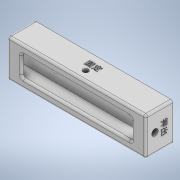
# Autodesk Inventor part: Part1
Saved by Autodesk Inventor 2021.4 (Build 254397000, 397)
## iProperties
Created: 2023-11-13
Part Number: Part1
Material: 一般
Document SubType Name: Modeling
Designer: ryusei
Density: 1 g/cm^3
Appearance: 既定
Author: ryusei
Autodesk Inventor part; units mm, degrees
ref_plane "YZ Plane" through (0, 0, 0) normal (1, 0, 0) x (0, 1, 0)
ref_plane "XZ Plane" through (0, 0, 0) normal (0, 1, 0) x (-1, 0, 0)
ref_plane "XY Plane" through (0, 0, 0) normal (0, 0, 1) x (1, 0, 0)
sketch "スケッチ1" plane through (0, 0, 0) normal (0, 0, 1) x (1, 0, 0)
  line L0 (-64, 17.5) -> (64, 17.5)
  line L1 (64, 17.5) -> (64, -17.5)
  line L2 (64, -17.5) -> (-64, -17.5)
  line L3 (-64, -17.5) -> (-64, 17.5)
  line L4 (-64, 17.5) -> (64, -17.5) construction
  line L5 (64, 17.5) -> (-64, -17.5) construction
  point P0 (0, 0)
  dimension "d0" = 128
  dimension "d1" = 35
  constraints: 12 end point, 2 midpoint, 2 parallel, 1 horizontal, 1 perpendicular
  measures "d0" distance of L1.end L2.end
  measures "d1" distance of L0.end L1.end
extrude "押し出し1" add sketch "スケッチ1" along normal blind 25
sketch "スケッチ3" plane through (-64, -17.5, 0) normal (-1, 0, 0) x (0, 0, 1)
  line L0 (10, 30) -> (23, 30)
  line L1 (23, 30) -> (23, 5)
  line L2 (23, 5) -> (10, 5)
  line L3 (10, 5) -> (10, 30)
  line L4 (0, 0) -> (25, 0) projected
  line L5 (25, 35) -> (25, 0) projected
  point P0 (0, 17.5)
  dimension "d8" = 13
  dimension "d9" = 25
  dimension "d10" = 5
  dimension "d11" = 2
  constraints: 8 end point, 2 parallel, 1 horizontal, 1 perpendicular
  measures "d8" distance of L1.end L2.end
  measures "d9" distance of L0.end L1.end
  measures "d10" distance between parallel lines of L4 L2
  measures "d11" distance between parallel lines of L5 L1
extrude "押し出し2" cut sketch "スケッチ3" against normal blind 118
sketch "スケッチ4" plane through (0, 0, 25) normal (0, 0, 1) x (1, 0, 0)
  line L0 (-51, 9.5) -> (51, 9.5)
  line L1 (51, 9.5) -> (51, -9.5)
  line L2 (51, -9.5) -> (-51, -9.5)
  line L3 (-51, -9.5) -> (-51, 9.5)
  line L4 (-51, 9.5) -> (51, -9.5) construction
  line L5 (51, 9.5) -> (-51, -9.5) construction
  point P0 (0, 0)
  dimension "d14" = 102
  dimension "d15" = 19
  constraints: 12 end point, 2 midpoint, 2 parallel, 1 horizontal, 1 perpendicular
  measures "d14" distance of L0.start L0.end
  measures "d15" distance of L0.end L1.end
extrude "押し出し3" cut sketch "スケッチ4" against normal blind 2
sketch "スケッチ6" plane through (64, -17.5, 0) normal (1, 0, 0) x (0, 0, -1)
  line L0 (0, 0) -> (-25, 0) projected
  line L1 (0, 0) -> (0, 35) projected
  line L2 (-25, 0) -> (-25, 35) projected
  point P0 (0, 17.5)
  point P1 (-16.5, 17.5)
  dimension "d27" = 17.5
  dimension "d46" = 8.5
  measures "d27" distance from line of L0 point (-16.5, 17.5)
  measures "d46" distance from line of L2 point (-16.5, 17.5)
hole "穴2" at (64, 0, 16.5) direction (-1, 0, 0) diameter 6 end through all
sketch "スケッチ7" plane through (-64, 17.5, 0) normal (0, 1, 0) x (1, 0, 0)
  line L0 (128, 0) -> (0, 0) projected
  line L1 (128, 0) -> (128, -25) projected
  line L2 (128, -25) -> (0, -25) projected
  point P0 (64, 0)
  point P1 (64, -16.5)
  dimension "d37" = 64
  dimension "d45" = 8.5
  measures "d37" distance from line of L1 point (64, -16.5)
  measures "d45" distance from line of L2 point (64, -16.5)
hole "穴3" at (0, 17.5, 16.5) direction (0, -1, 0) diameter 4.9 depth 8
sketch "スケッチ8" plane through (-64, -12.5, 10) normal (0, 0, 1) x (1, 0, 0)
  point P0 (64, 12.5)
  point P1 (29, 12.5)
  point P2 (99, 12.5)
  dimension "d47" = 35
  dimension "d48" = 35
  measures "d47" distance of point (29, 12.5) point (64, 12.5)
  measures "d48" distance of point (99, 12.5) point (64, 12.5)
hole "穴4" at (-35, 0, 10) at (35, 0, 10) direction (0, 0, -1) diameter 6 depth 15 counterbore diameter 10 counterbore depth 6
fillet "フィレット1" radius 2 12 edges at (-64, 17.5, 12.5) (0, 17.5, 25) (0, -17.5, 25) (-64, -17.5, 12.5) (64, 17.5, 12.5) (-64, 0, 25) (64, 0, 25) (64, -17.5, 12.5) (-51, 9.5, 24) (-51, -9.5, 24) (51, -9.5, 24) (51, 9.5, 24)
fillet "フィレット2" radius 2 8 edges at (50.4142, 8.9142, 25) (51, 0, 25) (50.4142, -8.9142, 25) (0, -9.5, 25) (-50.4142, -8.9142, 25) (-51, 0, 25) (-50.4142, 8.9142, 25) (0, 9.5, 25)
sketch "スケッチ9" plane through (-62, 17.5, 0) normal (0, 1, 0) x (1, 0, 0)
  line L0 (59.5, -8.4717) -> (64.5, -8.4717) construction
  line L1 (64.5, -8.4717) -> (64.5, -10) construction
  line L2 (64.5, -10) -> (59.5, -10) construction
  line L3 (59.5, -10) -> (59.5, -8.4717) construction
  line L4 (0, -25) -> (124, -25) projected
  line L5 (-2, 0) -> (-2, -23) projected
  line L6 (56.3598, -11.9081) -> (56.3598, -12.2565)
  line L7 (56.3598, -12.2565) -> (55.8209, -12.2565)
  line L8 (55.8209, -12.2565) -> (55.8209, -6.4016)
  line L9 (55.8209, -6.4016) -> (61.3274, -6.4016)
  line L10 (61.3274, -6.4016) -> (61.3274, -12.1512)
  line L11 (61.3274, -12.1512) -> (60.7925, -12.1512)
  line L12 (60.7925, -12.1512) -> (60.7925, -11.9081)
  line L13 (60.7925, -11.9081) -> (56.3598, -11.9081)
  line L14 (56.3598, -11.3975) -> (60.7925, -11.3975)
  line L15 (60.7925, -11.3975) -> (60.7925, -6.9121)
  line L16 (60.7925, -6.9121) -> (56.3598, -6.9121)
  line L17 (56.3598, -6.9121) -> (56.3598, -11.3975)
  spline S0 degree 2 poles (58.8314, -7.1552) (59.0462, -7.1795) (58.8558, -7.3132) knots 0 0 0 1 1 1
  line L18 (58.8558, -7.3132) -> (58.8558, -7.7468)
  line L19 (58.8558, -7.7468) -> (60.4684, -7.7468)
  line L20 (60.4684, -7.7468) -> (60.4684, -8.2533)
  line L21 (60.4684, -8.2533) -> (58.8558, -8.2533)
  line L22 (58.8558, -8.2533) -> (58.8558, -8.9786)
  line L23 (58.8558, -8.9786) -> (59.9579, -8.9786)
  line L24 (59.9579, -8.9786) -> (59.9579, -10.9964)
  line L25 (59.9579, -10.9964) -> (59.423, -10.9964)
  line L26 (59.423, -10.9964) -> (59.423, -10.7249)
  line L27 (59.423, -10.7249) -> (57.7577, -10.7249)
  line L28 (57.7577, -10.7249) -> (57.7577, -11.0774)
  line L29 (57.7577, -11.0774) -> (57.2188, -11.0774)
  line L30 (57.2188, -11.0774) -> (57.2188, -8.9786)
  line L31 (57.2188, -8.9786) -> (58.3209, -8.9786)
  line L32 (58.3209, -8.9786) -> (58.3209, -8.2533)
  line L33 (58.3209, -8.2533) -> (56.6556, -8.2533)
  line L34 (56.6556, -8.2533) -> (56.6556, -7.7468)
  line L35 (56.6556, -7.7468) -> (58.3209, -7.7468)
  line L36 (58.3209, -7.7468) -> (58.3209, -7.1552)
  line L37 (58.3209, -7.1552) -> (58.8314, -7.1552)
  line L38 (57.7577, -10.2954) -> (59.423, -10.2954)
  line L39 (59.423, -10.2954) -> (59.423, -9.4121)
  line L40 (59.423, -9.4121) -> (57.7577, -9.4121)
  line L41 (57.7577, -9.4121) -> (57.7577, -10.2954)
  spline S1 degree 2 poles (62.4579, -11.827) (63.7747, -11.0207) (63.7464, -9.25) knots 0 0 0 1 1 1
  line L42 (63.7464, -9.25) -> (64.3622, -9.3554)
  spline S2 degree 2 poles (64.3622, -9.3554) (64.4433, -9.4364) (64.3096, -9.5175) knots 0 0 0 1 1 1
  line L43 (64.3096, -9.5175) -> (64.1759, -10.4858)
  spline S3 degree 2 poles (64.1759, -10.4858) (64.577, -10.968) (65.2212, -11.3165) knots 0 0 0 1 1 1
  line L44 (65.2212, -11.3165) -> (65.2212, -8.7111)
  line L45 (65.2212, -8.7111) -> (63.3979, -8.7111)
  line L46 (63.3979, -8.7111) -> (63.3979, -8.2006)
  line L47 (63.3979, -8.2006) -> (67.4538, -8.2006)
  line L48 (67.4538, -8.2006) -> (67.4538, -8.7111)
  line L49 (67.4538, -8.7111) -> (65.7601, -8.7111)
  line L50 (65.7601, -8.7111) -> (65.7601, -9.7038)
  line L51 (65.7601, -9.7038) -> (67.6402, -9.7038)
  line L52 (67.6402, -9.7038) -> (67.6402, -10.2144)
  line L53 (67.6402, -10.2144) -> (65.7601, -10.2144)
  line L54 (65.7601, -10.2144) -> (65.7601, -11.5069)
  spline S4 degree 2 poles (65.7601, -11.5069) (66.1613, -11.6123) (66.5665, -11.6123) knots 0 0 0 1 1 1
  line L55 (66.5665, -11.6123) -> (68.3371, -11.6123)
  line L56 (68.3371, -11.6123) -> (68.2318, -12.1228)
  line L57 (68.2318, -12.1228) -> (66.5665, -12.1228)
  spline S5 degree 2 poles (66.5665, -12.1228) (65.0065, -12.1228) (64.0138, -10.9964) knots 0 0 0 1 1 1
  spline S6 degree 2 poles (64.0138, -10.9964) (63.6126, -11.8797) (62.8874, -12.3376) knots 0 0 0 1 1 1
  line L58 (62.8874, -12.3376) -> (62.4579, -11.827)
  line L59 (65.7318, -6.9121) -> (68.2034, -6.9121)
  line L60 (68.2034, -6.9121) -> (68.2034, -8.3343)
  line L61 (68.2034, -8.3343) -> (67.6686, -8.3343)
  line L62 (67.6686, -8.3343) -> (67.6686, -7.4226)
  line L63 (67.6686, -7.4226) -> (63.2075, -7.4226)
  line L64 (63.2075, -7.4226) -> (63.2075, -8.391)
  line L65 (63.2075, -8.391) -> (62.6726, -8.391)
  line L66 (62.6726, -8.391) -> (62.6726, -6.9121)
  line L67 (62.6726, -6.9121) -> (65.1159, -6.9121)
  line L68 (65.1159, -6.9121) -> (65.1159, -6.1341)
  line L69 (65.1159, -6.1341) -> (65.7075, -6.1341)
  spline S7 degree 2 poles (65.7075, -6.1341) (65.9749, -6.1868) (65.7318, -6.3489) knots 0 0 0 1 1 1
  line L70 (65.7318, -6.3489) -> (65.7318, -6.9121)
  point P0 (62, 0)
  dimension "d58" = 5
  dimension "d59" = 15
  dimension "d60" = 61.5
  constraints: 2 other
  measures "d58" distance of L0.start L0.end
  measures "d59" distance between parallel lines of L4 L2
  measures "d60" distance between parallel lines of L3 L5
extrude "押し出し4" cut sketch "スケッチ9" against normal blind 1
sketch "スケッチ10" plane through (64, -15.5, 0) normal (1, 0, 0) x (0, 0, -1)
  line L0 (-9.1711, 16.083) -> (-9.1711, 16.6219)
  line L1 (-9.1711, 16.6219) -> (-8.8227, 16.6219)
  line L2 (-8.8227, 16.6219) -> (-8.8227, 17.5336)
  line L3 (-8.8227, 17.5336) -> (-10.8932, 17.5336)
  line L4 (-10.8932, 17.5336) -> (-10.8932, 18.0725)
  line L5 (-10.8932, 18.0725) -> (-8.8227, 18.0725)
  line L6 (-8.8227, 18.0725) -> (-8.8227, 18.9598)
  line L7 (-8.8227, 18.9598) -> (-9.3332, 18.9598)
  line L8 (-9.3332, 18.9598) -> (-9.3332, 19.4947)
  line L9 (-9.3332, 19.4947) -> (-5.1436, 19.4947)
  line L10 (-5.1436, 19.4947) -> (-5.1436, 16.083)
  line L11 (-5.1436, 16.083) -> (-9.1711, 16.083)
  spline S0 degree 2 poles (-8.6079, 20.9452) (-8.6889, 21.241) (-8.8227, 21.5895) knots 0 0 0 1 1 1
  spline S1 degree 2 poles (-8.8227, 21.5895) (-9.0658, 21.7273) (-8.9037, 21.7799) knots 0 0 0 1 1 1
  line L12 (-8.9037, 21.7799) -> (-8.3121, 21.942)
  spline S2 degree 2 poles (-8.3121, 21.942) (-8.2311, 21.5895) (-8.0447, 20.9452) knots 0 0 0 1 1 1
  line L13 (-8.0447, 20.9452) -> (-6.4847, 20.9452)
  line L14 (-6.4847, 20.9452) -> (-6.4847, 21.8853)
  line L15 (-6.4847, 21.8853) -> (-5.9742, 21.8853)
  line L16 (-5.9742, 21.8853) -> (-5.9742, 20.9452)
  line L17 (-5.9742, 20.9452) -> (-4.7667, 20.9452)
  line L18 (-4.7667, 20.9452) -> (-4.7667, 20.4347)
  spline S3 degree 2 poles (-4.7667, 20.4347) (-4.7667, 20.2483) (-4.9288, 20.4104) knots 0 0 0 1 1 1
  line L19 (-4.9288, 20.4104) -> (-5.9742, 20.4104)
  line L20 (-5.9742, 20.4104) -> (-5.9742, 19.7094)
  line L21 (-5.9742, 19.7094) -> (-6.4847, 19.7094)
  line L22 (-6.4847, 19.7094) -> (-6.4847, 20.4104)
  line L23 (-6.4847, 20.4104) -> (-7.8826, 20.4104)
  spline S4 degree 2 poles (-7.8826, 20.4104) (-7.7773, 20.0619) (-7.6679, 19.7662) knots 0 0 0 1 1 1
  line L24 (-7.6679, 19.7662) -> (-8.1501, 19.6568)
  spline S5 degree 2 poles (-8.1501, 19.6568) (-8.2595, 19.9809) (-8.4215, 20.4104) knots 0 0 0 1 1 1
  line L25 (-8.4215, 20.4104) -> (-10.488, 20.4104)
  spline S6 degree 2 poles (-10.488, 20.4104) (-10.9175, 20.4104) (-10.9175, 20.8399) knots 0 0 0 1 1 1
  line L26 (-10.9175, 20.8399) -> (-10.9175, 21.3504)
  line L27 (-10.9175, 21.3504) -> (-10.4069, 21.4558)
  line L28 (-10.4069, 21.4558) -> (-10.4069, 21.0546)
  spline S7 degree 2 poles (-10.4069, 21.0546) (-10.4069, 20.9452) (-10.3016, 20.9452) knots 0 0 0 1 1 1
  line L29 (-10.3016, 20.9452) -> (-8.6079, 20.9452)
  line L30 (-6.7562, 16.6219) -> (-5.6541, 16.6219)
  line L31 (-5.6541, 16.6219) -> (-5.6541, 17.5336)
  line L32 (-5.6541, 17.5336) -> (-6.7562, 17.5336)
  line L33 (-6.7562, 17.5336) -> (-6.7562, 16.6219)
  line L34 (-6.7562, 18.9598) -> (-6.7562, 18.0725)
  line L35 (-6.7562, 18.0725) -> (-5.6541, 18.0725)
  line L36 (-5.6541, 18.0725) -> (-5.6541, 18.9598)
  line L37 (-5.6541, 18.9598) -> (-6.7562, 18.9598)
  line L38 (-8.3121, 16.6219) -> (-7.2667, 16.6219)
  line L39 (-7.2667, 16.6219) -> (-7.2667, 17.5336)
  line L40 (-7.2667, 17.5336) -> (-8.3121, 17.5336)
  line L41 (-8.3121, 17.5336) -> (-8.3121, 16.6219)
  line L42 (-8.3121, 18.9598) -> (-8.3121, 18.0725)
  line L43 (-8.3121, 18.0725) -> (-7.2667, 18.0725)
  line L44 (-7.2667, 18.0725) -> (-7.2667, 18.9598)
  line L45 (-7.2667, 18.9598) -> (-8.3121, 18.9598)
  spline S8 degree 2 poles (-5.492, 13.9355) (-5.5204, 13.7208) (-5.6541, 13.9112) knots 0 0 0 1 1 1
  line L46 (-5.6541, 13.9112) -> (-7.1047, 13.9112)
  line L47 (-7.1047, 13.9112) -> (-7.1047, 12.3229)
  line L48 (-7.1047, 12.3229) -> (-4.9572, 12.3229)
  line L49 (-4.9572, 12.3229) -> (-4.9572, 11.8123)
  spline S9 degree 2 poles (-4.9572, 11.8123) (-4.9815, 11.5976) (-5.1152, 11.788) knots 0 0 0 1 1 1
  line L50 (-5.1152, 11.788) -> (-7.1047, 11.788)
  line L51 (-7.1047, 11.788) -> (-7.1047, 10.2281)
  line L52 (-7.1047, 10.2281) -> (-5.5204, 10.2281)
  line L53 (-5.5204, 10.2281) -> (-5.5204, 9.7175)
  spline S10 degree 2 poles (-5.5204, 9.7175) (-5.5447, 9.5028) (-5.6825, 9.6932) knots 0 0 0 1 1 1
  line L54 (-5.6825, 9.6932) -> (-7.8583, 9.6932)
  line L55 (-7.8583, 9.6932) -> (-7.8583, 10.2281)
  line L56 (-7.8583, 10.2281) -> (-7.6152, 10.2281)
  line L57 (-7.6152, 10.2281) -> (-7.6152, 11.788)
  line L58 (-7.6152, 11.788) -> (-9.9248, 11.788)
  line L59 (-9.9248, 11.788) -> (-9.9248, 10.0133)
  line L60 (-9.9248, 10.0133) -> (-8.2878, 10.0133)
  line L61 (-8.2878, 10.0133) -> (-8.2878, 9.5028)
  spline S11 degree 2 poles (-8.2878, 9.5028) (-8.3121, 9.288) (-8.4458, 9.4785) knots 0 0 0 1 1 1
  line L62 (-8.4458, 9.4785) -> (-10.7311, 9.4785)
  line L63 (-10.7311, 9.4785) -> (-10.7311, 10.0133)
  line L64 (-10.7311, 10.0133) -> (-10.4353, 10.0133)
  line L65 (-10.4353, 10.0133) -> (-10.4353, 14.1786)
  line L66 (-10.4353, 14.1786) -> (-10.8121, 14.1786)
  line L67 (-10.8121, 14.1786) -> (-10.8121, 14.7135)
  line L68 (-10.8121, 14.7135) -> (-8.2595, 14.7135)
  line L69 (-8.2595, 14.7135) -> (-8.2595, 14.2029)
  spline S12 degree 2 poles (-8.2595, 14.2029) (-8.2878, 13.9882) (-8.4215, 14.1786) knots 0 0 0 1 1 1
  line L70 (-8.4215, 14.1786) -> (-9.9248, 14.1786)
  line L71 (-9.9248, 14.1786) -> (-9.9248, 12.3229)
  line L72 (-9.9248, 12.3229) -> (-7.6152, 12.3229)
  line L73 (-7.6152, 12.3229) -> (-7.6152, 13.9112)
  line L74 (-7.6152, 13.9112) -> (-7.911, 13.9112)
  line L75 (-7.911, 13.9112) -> (-7.911, 14.4461)
  line L76 (-7.911, 14.4461) -> (-5.492, 14.4461)
  line L77 (-5.492, 14.4461) -> (-5.492, 13.9355)
  point P0 (0, 15.5)
  point P1 (-7.8421, 15.4671)
  constraints: 1 other
extrude "押し出し5" cut sketch "スケッチ10" against normal blind 1
